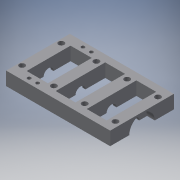
# Autodesk Inventor part: frame 1
Saved by Autodesk Inventor 2017 SP1 (Build 210196100, 196)
## iProperties
Created: 2017-06-14
Part Number: frame 1
Material: Generic
Document SubType Name: Modeling
Designer: RMcComber
Density: 1 g/cm^3
Appearance: Default
Author: RMcComber
Autodesk Inventor part; units mm, degrees
ref_plane "YZ Plane" through (0, 0, 0) normal (1, 0, 0) x (0, 1, 0)
ref_plane "XZ Plane" through (0, 0, 0) normal (0, 1, 0) x (-1, 0, 0)
ref_plane "XY Plane" through (0, 0, 0) normal (0, 0, 1) x (1, 0, 0)
sketch "Sketch1" plane through (0, 0, 0) normal (0, 0, 1) x (1, 0, 0)
  line L0 (51, -45) -> (-51, -45)
  line L1 (-51, -45) -> (-51, 45)
  line L2 (-51, 45) -> (51, 45)
  line L3 (51, 45) -> (51, -45)
  line L4 (51, -45) -> (-51, 45) construction
  line L5 (-51, -45) -> (51, 45) construction
  line L6 (-22, 0) -> (22, 0) construction
  line L7 (-36, 35) -> (-8, 35)
  line L8 (-8, 35) -> (-8, -35)
  line L9 (-8, -35) -> (-36, -35)
  line L10 (-36, -35) -> (-36, 35)
  line L11 (-36, 35) -> (-8, -35) construction
  line L12 (-8, 35) -> (-36, -35) construction
  line L13 (36, 35) -> (8, 35)
  line L14 (8, 35) -> (8, -35)
  line L15 (8, -35) -> (36, -35)
  line L16 (36, -35) -> (36, 35)
  line L17 (36, 35) -> (8, -35) construction
  line L18 (8, 35) -> (36, -35) construction
  point P0 (0, 0)
  point P1 (0, 0)
  dimension "d0" = 16
  dimension "d1" = 28
  dimension "d2" = 28
  dimension "d3" = 70
  dimension "d4" = 10
  dimension "d5" = 15
  constraints: 38 end point, 8 midpoint, 7 parallel, 4 perpendicular, 3 horizontal
  measures "d0" distance between parallel lines of L14 L8
  measures "d1" distance of L7.start L7.end
  measures "d2" distance of L13.start L13.end
  measures "d3" distance of L15.end L13.start
  measures "d4" distance between parallel lines of L7 L2
  measures "d5" distance between parallel lines of L1 L10
extrude "Extrusion1" add sketch "Sketch1" along normal blind 19
sketch "Sketch2" plane through (51, -45, 0) normal (1, 0, 0) x (0, 0, -1)
  circle A0 centre (0, 45) radius 7
  point P0 (0, 45)
  dimension "d8" = 14
  constraints: 1 centre point, 1 coincident
  measures "d8" diameter of A0
extrude "Extrusion2" cut sketch "Sketch2" against normal through all
sketch "Sketch3" plane through (51, -45, 19) normal (1, 0, 0) x (0, 0, -1)
  arc A0 (19, 52) -> (19, 38) centre (19, 45) ccw projected
  circle A1 centre (19, 45) radius 18
  dimension "d11" = 36
  constraints: 1 centre point, 1 coincident
  measures "d11" diameter of A1
extrude "Extrusion3" cut sketch "Sketch3" against normal blind 11
sketch "Sketch4" plane through (-51, -45, 19) normal (-1, 0, 0) x (0, 0, 1)
  arc A0 (-19, 38) -> (-19, 52) centre (-19, 45) ccw projected
  circle A1 centre (-19, 45) radius 17.5
  dimension "d14" = 35
  constraints: 1 centre point, 1 coincident
  measures "d14" diameter of A1
extrude "Extrusion4" cut sketch "Sketch4" against normal blind 11
sketch "Sketch5" plane through (-8, -35, 19) normal (-1, 0, 0) x (0, 0, 1)
  arc A0 (-19, 28) -> (-19, 42) centre (-19, 35) ccw projected
  circle A1 centre (-19, 35) radius 17.5
  dimension "d17" = 35
  constraints: 1 centre point, 1 coincident
  measures "d17" diameter of A1
extrude "Extrusion5" cut sketch "Sketch5" against normal blind 11
sketch "Sketch6" plane through (8, -35, 19) normal (1, 0, 0) x (0, 0, -1)
  arc A0 (19, 42) -> (19, 28) centre (19, 35) ccw projected
  circle A1 centre (19, 35) radius 17.5
  dimension "d20" = 35
  constraints: 1 centre point, 1 coincident
  measures "d20" diameter of A1
extrude "Extrusion6" [suppressed]
sketch "Sketch7" plane through (0, 0, 19) normal (0, 0, 1) x (1, 0, 0)
  line L0 (-36, -35) -> (-36, 35) projected
  line L1 (-51, 45) -> (-51, -45) projected
  line L2 (0, 30) -> (0, -30) construction
  circle A0 centre (0, 30) radius 4
  circle A1 centre (0, -30) radius 4
  line L3 (43.5, -30) -> (-43.5, -30) construction
  line L4 (-43.5, -30) -> (-43.5, 30) construction
  line L5 (-43.5, 30) -> (43.5, 30) construction
  line L6 (43.5, 30) -> (43.5, -30) construction
  line L7 (43.5, -30) -> (-43.5, 30) construction
  line L8 (-43.5, -30) -> (43.5, 30) construction
  circle A2 centre (-43.5, 30) radius 4
  circle A3 centre (-43.5, -30) radius 4
  circle A4 centre (43.5, -30) radius 4
  circle A5 centre (43.5, 30) radius 4
  point P0 (0, 0)
  point P1 (0, 0)
  dimension "d23" = 60
  dimension "d24" = 8
  dimension "d25" = 7.5
  dimension "d26" = 87
  constraints: 14 end point, 7 coincident, 6 centre point, 5 equal radius, 4 midpoint, 3 parallel, 1 horizontal, 1 perpendicular
  measures "d23" distance of L2.start L2.end
  measures "d24" diameter of A0
  measures "d25" distance between parallel lines of L0 L4
  measures "d26" distance of L4.end L5.end
extrude "Extrusion7" cut sketch "Sketch7" against normal through all
sketch "Sketch8" plane through (0, 0, 19) normal (0, 0, 1) x (1, 0, 0)
  line L0 (-51, 45) -> (-81, 45)
  line L1 (-81, 45) -> (-81, 31)
  line L2 (-81, 31) -> (-51, 31)
  line L3 (-51, 31) -> (-51, 45)
  line L4 (-51, -45) -> (-81, -45)
  line L5 (-81, -45) -> (-81, -31)
  line L6 (-81, -31) -> (-51, -31)
  line L7 (-51, -31) -> (-51, -45)
  line L8 (-81, 45) -> (-96, 45)
  line L9 (-96, 45) -> (-96, -45)
  line L10 (-96, -45) -> (-81, -45)
  line L11 (-81, -45) -> (-81, 45)
  point P0 (0, 0)
  dimension "d29" = 14
  dimension "d30" = 15
  dimension "d31" = 30
  dimension "d41" = 31
  constraints: 24 end point, 6 parallel, 3 horizontal, 3 perpendicular, 1 collinear
  measures "d29" distance between parallel lines of L0 L2
  measures "d30" distance between parallel lines of L1 L9
  measures "d31" distance of L0.start L0.end
  measures "d41" distance from line of point (0, 0) L2
extrude "Extrusion8" add sketch "Sketch8" against normal up to surface (19 mm away)
sketch "Sketch9" plane through (-96, -45, 19) normal (-1, 0, 0) x (0, 0, 1)
  circle A0 centre (-19, 45) radius 17.5
  dimension "d34" = 35
  constraints: 1 centre point, 1 coincident
  measures "d34" diameter of A0
extrude "Extrusion9" cut sketch "Sketch9" against normal blind 11
sketch "Sketch10" plane through (0, 0, 0) normal (0, 0, -1) x (-1, 0, 0)
  line L0 (96, -17.5) -> (85, -17.5) projected
  circle A0 centre (43.5, 30) radius 4 projected
  circle A1 centre (0, 30) radius 4 projected
  circle A2 centre (-43.5, 30) radius 4 projected
  line L1 (85, 17.5) -> (96, 17.5) projected
  line L2 (96, 17.5) -> (96, 45) projected
  line L3 (96, 45) -> (-51, 45) projected
  line L4 (-51, 45) -> (-51, 18) projected
  line L5 (-51, 18) -> (-40, 18) projected
  line L6 (-40, 18) -> (-40, 7) projected
  line L7 (-40, 7) -> (-36, 7) projected
  line L8 (-36, 7) -> (-36, 35) projected
  line L9 (-36, 35) -> (-8, 35) projected
  line L10 (-8, -7) -> (-8, -35) projected
  line L11 (36, 7) -> (40, 7) projected
  line L12 (-3, 7) -> (-3, 17.5) projected
  line L13 (-3, 17.5) -> (8, 17.5) projected
  line L14 (8, 17.5) -> (8, 35) projected
  line L15 (8, 35) -> (36, 35) projected
  line L16 (36, 35) -> (36, 7) projected
  line L17 (40, 7) -> (40, 17.5) projected
  line L18 (40, 17.5) -> (51, 17.5) projected
  line L19 (51, 17.5) -> (51, 31) projected
  line L20 (51, 31) -> (81, 31) projected
  line L21 (81, 31) -> (81, -31) projected
  line L22 (90.5, 17.5) -> (90.5, 27.5) construction
  line L23 (91, -17.5) -> (91, -27.5) construction
  circle A3 centre (90.5, 27.5) radius 4
  circle A4 centre (91, -27.5) radius 4
  line L24 (96, -17.5) -> (85, -17.5) projected
  line L25 (81, -31) -> (51, -31) projected
  line L26 (51, -31) -> (51, -17.5) projected
  line L27 (51, -17.5) -> (40, -17.5) projected
  line L28 (40, -17.5) -> (40, -7) projected
  line L29 (40, -7) -> (36, -7) projected
  line L30 (36, -7) -> (36, -35) projected
  line L31 (36, -35) -> (8, -35) projected
  line L32 (8, -35) -> (8, -17.5) projected
  line L33 (8, -17.5) -> (-3, -17.5) projected
  line L34 (-3, -17.5) -> (-3, -7) projected
  line L35 (-3, -7) -> (-8, -7) projected
  line L36 (-8, -35) -> (-36, -35) projected
  line L37 (-36, -35) -> (-36, -7) projected
  line L38 (-36, -7) -> (-40, -7) projected
  line L39 (-40, -7) -> (-40, -18) projected
  line L40 (-40, -18) -> (-51, -18) projected
  line L41 (-51, -18) -> (-51, -45) projected
  line L42 (-51, -45) -> (96, -45) projected
  line L43 (96, -45) -> (96, -17.5) projected
  line L44 (-8, 35) -> (-8, 7) projected
  line L45 (-8, 7) -> (-3, 7) projected
  line L46 (85, -17.5) -> (85, 17.5) projected
  point P0 (86, -17.5)
  point P1 (0, 0)
  dimension "d37" = 8
  dimension "d38" = 10
  constraints: 4 end point, 3 parallel, 2 centre point, 2 coincident, 1 equal radius, 1 midpoint, 1 point on line
  measures "d37" diameter of A3
  measures "d38" distance of L22.start L22.end
extrude "Extrusion10" cut sketch "Sketch10" against normal through all contours A3 | A4
sketch "Sketch11" plane through (0, 0, 19) normal (0, 0, 1) x (1, 0, 0)
  circle A0 centre (-58.5, 38) radius 2.5 projected
  circle A1 centre (-70.5, 38) radius 2.5 projected
  circle A2 centre (-70.5, -38) radius 2.5 projected
  circle A3 centre (-58.5, -38) radius 2.5 projected
  point P0 (0, 0)
extrude "Extrusion11" cut sketch "Sketch11" against normal through all
sketch "Sketch12" plane through (-85, -45, 19) normal (-1, 0, 0) x (0, 0, 1)
  arc A0 (-19, 38) -> (-19, 52) centre (-19, 45) ccw projected
  line L0 (-19, 52) -> (-19, 38)
  line L1 (-19, 27.5) -> (-19, 62.5) projected
  point P0 (-19, 45)
  constraints: 2 end point, 1 collinear
extrude "Extrusion12" cut sketch "Sketch12" against normal blind 10
body "Solid1"
